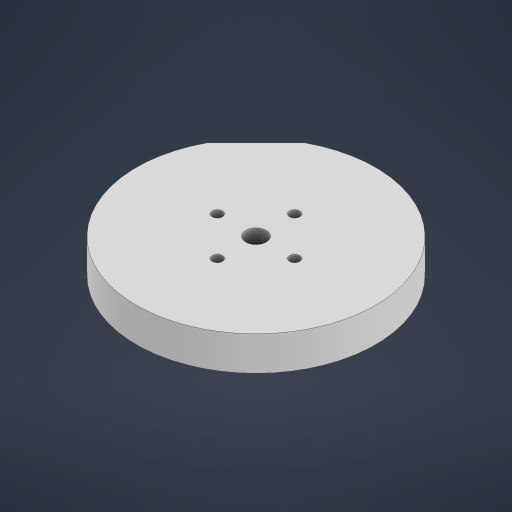
# Autodesk Inventor part: Pulley-35
Saved by Autodesk Inventor 2023 (Build 270158000, 158)
## iProperties
Created: 2023-09-04
Part Number: Pulley-35
Material: Generic
Document SubType Name: Modeling
Designer: Abhinav
Density: 1 g/cm^3
Appearance: Default
Author: Abhinav
Autodesk Inventor part; units mm, degrees
ref_plane "YZ Plane" through (0, 0, 0) normal (1, 0, 0) x (0, 1, 0)
ref_plane "XZ Plane" through (0, 0, 0) normal (0, 1, 0) x (-1, 0, 0)
ref_plane "XY Plane" through (0, 0, 0) normal (0, 0, 1) x (1, 0, 0)
sketch "Sketch1" plane through (0, 0, 0) normal (0, 1, 0) x (-1, 0, 0)
  arc A0 (30.7371, -16.74) -> (16.74, -30.7371) centre (0, 0) ccw
  line L0 (30.7371, -16.74) -> (16.74, -30.7371)
  circle A1 centre (11.3137, 0) radius 1.5
  line L1 (0, -11.3137) -> (11.3137, 0) construction
  line L2 (11.3137, 0) -> (0, 11.3137) construction
  circle A2 centre (0, -11.3137) radius 1.5
  circle A3 centre (0, 11.3137) radius 1.5
  line L3 (0, 11.3137) -> (-11.3137, 0) construction
  line L4 (-11.3137, 0) -> (0, -11.3137) construction
  line L5 (11.3137, 0) -> (-11.3137, 0) construction
  line L6 (0, -11.3137) -> (0, 11.3137) construction
  circle A4 centre (-11.3137, 0) radius 1.5
  circle A5 centre (0, 0) radius 3
  dimension "d2" = 70
  dimension "d13" = 16
  dimension "d14" = 3
  dimension "d16" = 6
  constraints: 14 end point, 6 centre point, 6 coincident, 3 equal radius, 2 parallel, 2 perpendicular, 2 point on circle, 1 midpoint
  measures "d2" diameter of A0
  measures "d13" distance of L3.end L2.end
  measures "d14" diameter of A2
  measures "d16" diameter of A5
extrude "Extrusion1" add sketch "Sketch1" along normal blind 10
sketch "Sketch3" plane through (-30.7371, 0, -16.74) normal (-0.7071, 0, -0.7071) x (-0.7071, 0, 0.7071)
  line L0 (-19.7949, 0) -> (0, 0) construction
  line L1 (-19.7949, 10) -> (0, 10) construction
  line L2 (0, 0) -> (-19.7949, 10) construction
  circle A0 centre (-9.8974, 5) radius 1.5
  point P0 (-9.8974, 0)
  dimension "d17" = 3
  constraints: 2 end point, 1 centre point, 1 midpoint
  measures "d17" diameter of A0
extrude "Extrusion3" add sketch "Sketch3" along normal blind 5
body "Solid1"
